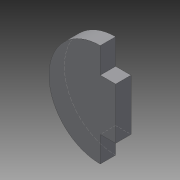
# Autodesk Inventor part: Cradel holder
Saved by Autodesk Inventor 2015 (Build 190159000, 159)
## iProperties
Created: 2014-11-13
Part Number: Cradel holder
Material: Generic
Document SubType Name: Modeling
Designer: karl
Density: 1 g/cm^3
Appearance: Default
Author: karl
Autodesk Inventor part; units mm, degrees
ref_plane "YZ Plane" through (0, 0, 0) normal (1, 0, 0) x (0, 1, 0)
ref_plane "XZ Plane" through (0, 0, 0) normal (0, 1, 0) x (-1, 0, 0)
ref_plane "XY Plane" through (0, 0, 0) normal (0, 0, 1) x (1, 0, 0)
sketch "Sketch1" plane through (0, 0, 0) normal (0, 1, 0) x (-1, 0, 0)
  circle A0 centre (0, 0) radius 10
  line L0 (0, -10) -> (0, 10)
  dimension "d0" = 20
  constraints: 2 end point, 2 point on circle, 1 centre point, 1 coincident, 1 midpoint, 1 vertical
  measures "d0" diameter of A0
extrude "Extrusion1" add sketch "Sketch1" along normal blind 3 contours A0 L0 picked at (2.6061, 2.0783)
sketch "Sketch2" plane through (0, 3, 0) normal (0, 1, 0) x (1, 0, 0)
  line L0 (0, 5) -> (3, 5)
  line L1 (3, 5) -> (3, -5)
  line L2 (3, -5) -> (0, -5)
  line L3 (0, -5) -> (0, 5)
  line L4 (0, -10) -> (0, 10) projected
  point P0 (0, 0)
  point P1 (3, 0)
  point P2 (0, 0)
  dimension "d3" = 3
  dimension "d4" = 10
  constraints: 8 end point, 2 midpoint, 2 parallel, 1 collinear, 1 horizontal, 1 horizontal alignment, 1 perpendicular
  measures "d3" distance of L1.end L2.end
  measures "d4" distance of L0.end L1.end
extrude "Extrusion2" add sketch "Sketch2" against normal blind 3
sketch "Sketch3" plane through (0, 3, 0) normal (0, 1, 0) x (1, 0, 0)
  circle A0 centre (-5, 0) radius 1.5
  line L0 (0, -10) -> (0, -5) projected
  point P0 (0, 0)
  dimension "d7" = 3
  dimension "d8" = 5
  constraints: 1 centre point, 1 horizontal alignment
  measures "d7" diameter of A0
  measures "d8" distance from line of A0.centre L0
extrude "Extrusion3" cut sketch "Sketch3" against normal blind 3
body "Solid1"
